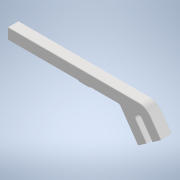
# Autodesk Inventor part: grip_N_fix
Saved by Autodesk Inventor 2021 (Build 250183000, 183)
## iProperties
Created: 2021-05-09
Part Number: grip_N_fix
Material: Generic
Document SubType Name: Modeling
Designer: Alsayaary
Density: 1 g/cm^3
Appearance: Default
Author: Abdulrahman
Autodesk Inventor part; units mm, degrees
ref_plane "YZ Plane" through (0, 0, 0) normal (1, 0, 0) x (0, 1, 0)
ref_plane "XZ Plane" through (0, 0, 0) normal (0, 1, 0) x (-1, 0, 0)
ref_plane "XY Plane" through (0, 0, 0) normal (0, 0, 1) x (1, 0, 0)
sketch "Sketch1" plane through (0, 0, 0) normal (0, 0, 1) x (1, 0, 0)
  line L0 (98.7752, 71.1622) -> (146.7319, 2.6729)
  line L1 (146.7319, 2.6729) -> (171.3065, 19.8802)
  line L2 (171.3065, 19.8802) -> (142.6276, 60.8378)
  arc A0 (156.364, 72.364) -> (142.6276, 60.8378) centre (150, 66) ccw
  line L3 (156.364, 72.364) -> (191.7193, 37.0086)
  line L4 (191.7193, 37.0086) -> (212.9325, 58.2218)
  line L5 (212.9325, 58.2218) -> (177.5772, 93.5772)
  arc A1 (177.5772, 93.5772) -> (150, 105) centre (150, 66) ccw
  line L6 (91.4028, 75) -> (-208.5972, 75)
  line L7 (150, 105) -> (-208.5972, 105)
  line L8 (-208.5972, 105) -> (-208.5972, 75)
  line L9 (0, 128.7567) -> (0, -18.341) projected
  line L10 (-292.9031, 0) -> (297.2384, 0) projected
  arc A2 (98.7752, 71.1622) -> (91.4028, 75) centre (91.4028, 66) ccw
  dimension "d38" = 30
  dimension "d39" = 30
  dimension "d40" = 9
  dimension "d47" = 30
  dimension "d53" = 9
  dimension "d56" = 300
  dimension "d58" = 150
  dimension "d59" = 50
  dimension "d60" = 35
  dimension "d61" = 75
  dimension "d88" = 45
  constraints: 18 end point, 6 perpendicular, 6 point on circle, 6 tangent, 3 centre point, 1 coincident, 1 parallel
  measures "d38" distance of L3.end L4.end
  measures "d39" distance of L0.end L1.end
  measures "d40" radius of A0
  measures "d47" distance of L7.end L6.end
  measures "d53" radius of A2
  measures "d56" distance of L6.start L6.end
  measures "d58" distance from line of L9 A0.centre
  measures "d59" distance from line of A0.centre L4
  measures "d60" angle of L1 L6
  measures "d61" distance between parallel lines of L10 L6
  measures "d88" angle of L6 L4
extrude "Extrusion1" add sketch "Sketch1" along normal mid plane 30
sketch "Sketch4" plane through (0, 0, 0) normal (0, 0, 1) x (1, 0, 0)
  line L0 (-208.5972, 75) -> (91.4028, 75) projected
  line L1 (-15, 75) -> (15, 75)
  line L2 (-15, 75) -> (-15, 74)
  line L3 (-15, 74) -> (15, 74)
  line L4 (15, 74) -> (15, 75)
  line L5 (0, 90) -> (0, -15) projected
  point P0 (0, 0)
  dimension "d62" = 30
  dimension "d63" = 15
  dimension "d64" = 1
  constraints: 8 end point, 2 perpendicular, 2 point on line, 1 vertical
  measures "d62" distance of L2.end L3.end
  measures "d63" distance between parallel lines of L5 L2
  measures "d64" distance of L3.end L1.end
extrude "Extrusion4" add sketch "Sketch4" along normal mid plane 30
fillet "Fillet1" radius 2 14 edges at (-111.7986, 75, 15) (95.5586, 73.9831, 15) (122.7535, 36.9176, 15) (53.2014, 75, 15) (-111.7986, 75, -15) (95.5586, 73.9831, -15) (122.7535, 36.9176, -15) (53.2014, 75, -15) (164.9247, 102.0313, -15) (195.2548, 75.8995, -15) (-29.2986, 105, -15) (164.9247, 102.0313, 15) (195.2548, 75.8995, 15) (-29.2986, 105, 15)
sketch "Sketch5" plane through (-208.5972, 77, -15) normal (-1, 0, 0) x (0, 0, 1)
  line L0 (27.5, 25.5) -> (2.5, 25.5)
  line L1 (2.5, 25.5) -> (2.5, 0.5)
  line L2 (2.5, 0.5) -> (27.5, 0.5)
  line L3 (27.5, 0.5) -> (27.5, 25.5)
  line L4 (2, 28) -> (28, 28) projected
  line L5 (0, 0) -> (0, 26) projected
  line L6 (2, -2) -> (28, -2) projected
  line L7 (30, 26) -> (30, 0) projected
  point P0 (15, -77)
  dimension "d68" = 2.5
  dimension "d69" = 2.5
  dimension "d70" = 2.5
  dimension "d71" = 2.5
  constraints: 8 end point, 2 parallel, 1 horizontal, 1 perpendicular
  measures "d68" distance between parallel lines of L0 L4
  measures "d69" distance between parallel lines of L5 L1
  measures "d70" distance between parallel lines of L6 L2
  measures "d71" distance between parallel lines of L7 L3
extrude "Extrusion5" cut sketch "Sketch5" against normal blind 350
fillet "Fillet2" radius 2 4 edges at (-33.5972, 77.5, 12.5) (-33.5972, 77.5, -12.5) (-33.5972, 102.5, -12.5) (-33.5972, 102.5, 12.5)
sketch "Sketch6" plane through (191.7193, 37.0086, -15) normal (0.7071068, -0.7071068, 0) x (0.7071068, 0.7071068, 0)
  line L0 (2.5, 27.5) -> (27.5, 27.5)
  line L1 (27.5, 27.5) -> (27.5, 2.5)
  line L2 (27.5, 2.5) -> (2.5, 2.5)
  line L3 (2.5, 2.5) -> (2.5, 27.5)
  line L4 (28, 0) -> (0, 0) projected
  line L5 (30, 2) -> (30, 28) projected
  line L6 (0, 30) -> (28, 30) projected
  line L7 (0, 0) -> (0, 30) projected
  point P0 (-161.7351, 15)
  dimension "d75" = 2.5
  dimension "d76" = 2.5
  dimension "d77" = 2.5
  dimension "d78" = 2.5
  constraints: 8 end point, 2 parallel, 1 horizontal, 1 perpendicular
  measures "d75" distance between parallel lines of L4 L2
  measures "d76" distance between parallel lines of L5 L1
  measures "d77" distance between parallel lines of L6 L0
  measures "d78" distance between parallel lines of L7 L3
extrude "Extrusion6" cut sketch "Sketch6" against normal blind 50
sketch "Sketch7" plane through (171.3065, 19.8802, -15) normal (0.5735764, -0.819152, 0) x (0.819152, 0.5735764, 0)
  line L0 (-27.5, 27.5) -> (-2.5, 27.5)
  line L1 (-2.5, 27.5) -> (-2.5, 2.5)
  line L2 (-2.5, 2.5) -> (-27.5, 2.5)
  line L3 (-27.5, 2.5) -> (-27.5, 27.5)
  line L4 (-28, 30) -> (0, 30) projected
  line L5 (0, 30) -> (0, 0) projected
  line L6 (0, 0) -> (-28, 0) projected
  line L7 (-30, 2) -> (-30, 28) projected
  point P0 (-151.7289, 15)
  dimension "d81" = 2.5
  dimension "d82" = 2.5
  dimension "d83" = 2.5
  dimension "d84" = 2.5
  constraints: 8 end point, 2 parallel, 1 horizontal, 1 perpendicular
  measures "d81" distance between parallel lines of L4 L0
  measures "d82" distance between parallel lines of L5 L1
  measures "d83" distance between parallel lines of L6 L2
  measures "d84" distance between parallel lines of L7 L3
extrude "Extrusion7" cut sketch "Sketch7" against normal blind 50
fillet "Fillet3" radius 2 14 edges at (174.0416, 54.6863, 15) (156.967, 40.359, 15) (144.2149, 72.8944, 15) (156.967, 40.359, -15) (174.0416, 54.6863, -15) (144.2149, 72.8944, -15) (134.4398, 24.5865, -12.5) (134.4398, 24.5865, 12.5) (154.9186, 38.9259, 12.5) (154.9186, 38.9259, -12.5) (175.8087, 56.4548, -12.5) (193.4864, 74.1324, -12.5) (193.4864, 74.1324, 12.5) (175.8087, 56.4548, 12.5)
equation "\"d39\" = d38"
equation "\"secure_arm_radii\" = 9"
equation "\"rack_tooth_thickness\" = 5"
equation "\"rack_tooth_addendum\" = 5"
equation "\"rack_tooth_dedendum\" = 5"
equation "\"hoop_bearing_length\" = 5deg"
equation "\"secure_arm_angle\" = 35deg"
equation "\"hoop_tabs_thickness\" = 6"
equation "\"hoop_tabs_hole\" = 12"
equation "\"support_baseClamp_thickness\" = 8"
equation "\"support_frame_endHoleBuffer\" = 25"
equation "\"support_frame_squareBarThickness\" = 5"
equation "\"support_baseClamp_sleeveSweepTerminationAngle\" = 55deg"
equation "\"support_baseClamp_sleeveHoleDiameter\" = 12"
equation "\"support_frame_squareBarFillet\" = 2"
equation "\"support_baseClamp_platformWidthBuffer\" = 0"
equation "\"support_baseClamp_platformThickness\" = 15"
equation "\"support_baseClamp_platformLengthBuffer\" = 35"
equation "\"hoop_angle_z\" = 45deg"
equation "\"hoop_cable_diam\" = 5"
equation "\"hoop_cable_pulley_diam\" = 22"
equation "\"wheelchair_deployed_width\" = 635"
equation "\"wheelchair_deployed_height\" = 914"
equation "\"wheelchair_deployed_length\" = 1067"
equation "\"sm_varx_pinPlate_thickness\" = 5"
equation "\"sm_varx_member_tolerance\" = 0.5"
equation "\"sm_varx_pinPlate_holeDiameter\" = 5"
equation "\"sm_varx_squareBarThickness\" = 2.5"
body "Solid1"
